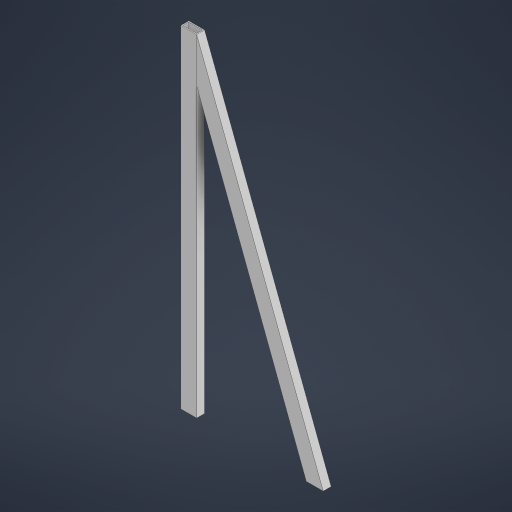
# Autodesk Inventor part: Part1
Saved by Autodesk Inventor 2023 (Build 270158000, 158)
## iProperties
Created: 2023-01-08
Part Number: Part1
Material: Generic
Document SubType Name: Modeling
Designer: Terrence
Density: 1 g/cm^3
Appearance: Default
Author: Terrence
Autodesk Inventor part; units mm, degrees
ref_plane "YZ Plane" through (0, 0, 0) normal (1, 0, 0) x (0, 1, 0)
ref_plane "XZ Plane" through (0, 0, 0) normal (0, 1, 0) x (-1, 0, 0)
ref_plane "XY Plane" through (0, 0, 0) normal (0, 0, 1) x (1, 0, 0)
sketch "Sketch1" plane through (0, 0, 0) normal (0, 1, 0) x (-1, 0, 0)
  line L0 (0, 0) -> (50.8, 0)
  line L1 (50.8, 0) -> (50.8, -25.4)
  line L2 (50.8, -25.4) -> (0, -25.4)
  line L3 (0, -25.4) -> (0, 0)
  dimension "d0" = 50.8
  dimension "d1" = 25.4
  constraints: 8 end point, 2 parallel, 1 horizontal, 1 perpendicular
  measures "d0" distance of L1.end L2.end
  measures "d1" distance of L0.end L1.end
extrude "Extrusion1" add sketch "Sketch1" along normal blind 1066.8
shell "Shell1" thickness 3.175 removed faces 2 at (-16.9333, 0, -16.9333) at (-16.9333, 1066.8, -16.9333)
sketch "Sketch2" plane through (-50.8, 0, 0) normal (0, 0, 1) x (1, 0, 0)
  line L0 (457.2, 0) -> (50.8, 1066.8)
  line L1 (402.8387, 0) -> (50.8, 924.1015)
  line L2 (50.8, 0) -> (50.8, 1066.8) projected
  line L3 (50.8, 0) -> (457.2, 0)
  point P0 (50.8, 1058.5302)
  dimension "d6" = 50.8
  dimension "d7" = 406.4
  constraints: 6 end point, 2 point on line, 1 horizontal
  measures "d6" distance between parallel lines of L0 L1
  measures "d7" distance of L2.start L0.start
extrude "Extrusion2" add sketch "Sketch2" against normal up to surface (25.4 mm away) separate body contours L3 L1 L2 L0
body "Solid1"
body "Solid2"
